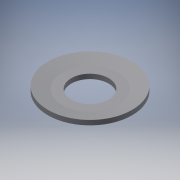
# Autodesk Inventor part: PODKŁADKA M8X18
Saved by Autodesk Inventor 2017 SP1 (Build 210196100, 196)
## iProperties
Created: 2021-01-06
Part Number: PODKŁADKA M8X18
Material: Stal
Document SubType Name: Modeling
Designer: Napoleon
Mass: 1.603 g
Surface Area: 4.95688 cm^2
Volume: 0.204204 cm^3
Density: 7.85 g/cm^3
Appearance: Anodowany - brązowy
Author: Napoleon
Autodesk Inventor part; units mm, degrees
ref_plane "YZ Plane" through (0, 0, 0) normal (1, 0, 0) x (0, 1, 0)
ref_plane "XZ Plane" through (0, 0, 0) normal (0, 1, 0) x (-1, 0, 0)
ref_plane "XY Plane" through (0, 0, 0) normal (0, 0, 1) x (1, 0, 0)
sketch "Szkic1" plane through (0, 0, 0) normal (0, 1, 0) x (-1, 0, 0)
  line L0 (-4, 0) -> (-4, 1)
  line L1 (-4, 0) -> (-6, 0)
  line L2 (-9, 1.6) -> (-9, 0.6)
  line L3 (-9, 0.6) -> (-6, 0)
  line L4 (-4, 1) -> (-6, 1)
  line L5 (-6, 1) -> (-9, 1.6)
  line L6 (0, 0) -> (0, 1.6)
  constraints: 14 end point, 2 horizontal, 2 vertical, 1 perpendicular
revolve "Obrót1" add sketch "Szkic1" angle 360 about axis through (0, 0, 0) along (0, 0, 1)
